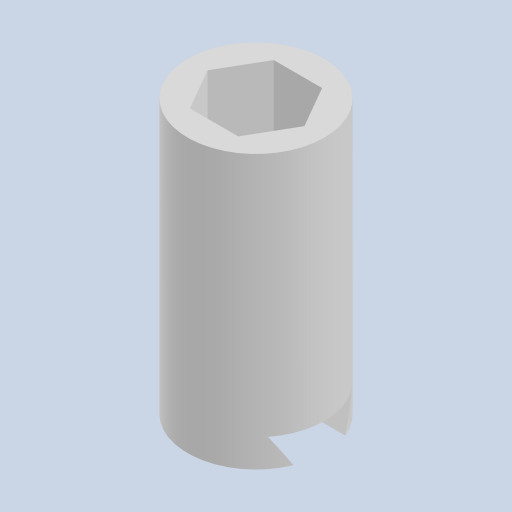
# Autodesk Inventor part: Varf Biti
Saved by Autodesk Inventor 2024 (Build 280153000, 153)
## iProperties
Created: 2024-04-20
Part Number: Varf Biti
Material: Generic
Document SubType Name: Modeling
Designer: mirun
Density: 1 g/cm^3
Appearance: Default
Author: mirun
Autodesk Inventor part; units mm, degrees
ref_plane "YZ Plane" through (0, 0, 0) normal (1, 0, 0) x (0, 1, 0)
ref_plane "XZ Plane" through (0, 0, 0) normal (0, 1, 0) x (-1, 0, 0)
ref_plane "XY Plane" through (0, 0, 0) normal (0, 0, 1) x (1, 0, 0)
sketch "Sketch1" plane through (0, 0, 0) normal (0, 1, 0) x (-1, 0, 0)
  circle A0 centre (0, 0) radius 5.5
  dimension "d0" = 11
  constraints: 1 centre point, 1 coincident
  measures "d0" diameter of A0
extrude "Extrusion1" add sketch "Sketch1" along normal blind 8
sketch "Sketch2" plane through (0, 0, 0) normal (1, 0, 0) x (0, 1, 0)
  line L0 (0, 0) -> (2.7456, 0)
  line L1 (2.25, 0) -> (2.25, 3.375)
  line L2 (2.25, 3.375) -> (0, 2.076)
  line L3 (0, -5.5) -> (0, 5.5) construction
  line L4 (2.25, 0) -> (2.25, -3.375)
  line L5 (2.25, -3.375) -> (0, -2.076)
  line L6 (0, -2.076) -> (0, 2.076)
  dimension "d9" = 3.375
  dimension "d10" = 2.25
  dimension "d11" = 60
  constraints: 12 end point, 2 point on line, 2 symmetric about line, 2 vertical, 1 horizontal
  measures "d9" distance of L1.start L1.end
  measures "d10" distance from line of L0.start L1
  measures "d11" angle of L2 L1
extrude "Extrusion2" cut sketch "Sketch2" along normal through all both and the other way through all
sketch "Sketch3" plane through (0, 8, 0) normal (0, 1, 0) x (1, 0, 0)
  circle A0 centre (0, 0) radius 5.5 projected
  line L0 (1.9486, 3.375) -> (3.8971, 0)
  line L1 (3.8971, 0) -> (1.9486, -3.375)
  line L2 (1.9486, -3.375) -> (-1.9486, -3.375)
  line L3 (-1.9486, -3.375) -> (-3.8971, 0)
  line L4 (-3.8971, 0) -> (-1.9486, 3.375)
  line L5 (-1.9486, 3.375) -> (1.9486, 3.375)
  circle A1 centre (0, 0) radius 2.625
  dimension "d14" = 6.75
  dimension "d15" = 5.25
  constraints: 12 end point, 2 coincident, 1 centre point, 13 other
  measures "d14" distance between parallel lines of L2 L5
  measures "d15" diameter of A1
extrude "Extrusion3" cut sketch "Sketch3" against normal blind 2.5 contours A1
extrude "Extrusion4" add sketch "Sketch3" along normal blind 14 contours A0
body "Solid1"
